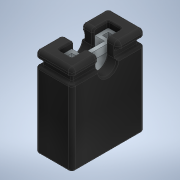
# Autodesk Inventor part: PinHeaderJumper
Saved by Autodesk Inventor 2021 (Build 250183000, 183)
## iProperties
Created: 2021-09-29
Part Number: PinHeaderJumper
Material: Generic
Document SubType Name: Modeling
Designer: ermoz
Density: 1 g/cm^3
Appearance: Default
Author: ermoz
Autodesk Inventor part; units mm, degrees
ref_plane "YZ Plane" through (0, 0, 0) normal (1, 0, 0) x (0, 1, 0)
sketch "Sketch1" plane through (0, 0, 0) normal (0, 1, 0) x (-1, 0, 0)
  line L0 (1.27, 2.54) -> (-1.27, 2.54)
  line L1 (-1.27, 2.54) -> (-1.27, -2.54)
  line L2 (-1.27, -2.54) -> (1.27, -2.54)
  line L3 (1.27, -2.54) -> (1.27, 2.54)
  line L4 (1.27, 2.54) -> (-1.27, -2.54) construction
  line L5 (-1.27, 2.54) -> (1.27, -2.54) construction
  line L6 (0.47, 1.74) -> (-0.47, 1.74)
  line L7 (-0.47, 1.74) -> (-0.47, -1.74)
  line L8 (-0.47, -1.74) -> (0.47, -1.74)
  line L9 (0.47, -1.74) -> (0.47, 1.74)
  point P0 (0, 0)
  dimension "d0" = 2.54
  dimension "d1" = 5.08
  dimension "d2" = 0.8
  constraints: 20 end point, 4 parallel, 2 midpoint, 2 perpendicular, 1 horizontal, 3 other
  measures "d0" distance of L2.end L1.end
  measures "d1" distance of L0.end L1.end
  measures "d2" distance between parallel lines of L3 L9
extrude "Extrusion1" add sketch "Sketch1" along normal blind 6.2
sketch "Sketch2" plane through (1.27, 0, 2.54) normal (1, 0, 0) x (0, 0, -1)
  line L0 (3.19, 5.2) -> (1.89, 5.2)
  line L1 (1.89, 5.2) -> (1.89, 7.2)
  line L2 (1.89, 7.2) -> (3.19, 7.2)
  line L3 (3.19, 7.2) -> (3.19, 5.2)
  line L4 (0, 6.2) -> (5.08, 6.2) projected
  line L5 (3.19, 5.2) -> (1.89, 7.2) construction
  line L6 (1.89, 5.2) -> (3.19, 7.2) construction
  circle A0 centre (2.54, 5.2) radius 0.65
  point P0 (2.54, 0)
  point P1 (2.54, 6.2)
  point P2 (3.19, 6.2)
  point P3 (1.89, 6.2)
  dimension "d5" = 1.3
  dimension "d6" = 2
  constraints: 12 end point, 4 midpoint, 2 parallel, 1 horizontal, 1 perpendicular, 3 other
  measures "d5" distance of L1.end L2.end
  measures "d6" distance of L2.end L0.start
extrude "Extrusion2" cut sketch "Sketch2" against normal through all contours A0 L0 | A0 L1 L4 L3 | L0 A0
ref_plane "Work Plane1" through (0, 5.7, 0) normal (0, 1, 0) x (1, 0, 0)
sketch "Sketch3" plane through (0, 5.7, 0) normal (0, 1, 0) x (1, 0, 0)
  line L0 (1.27, -2.54) -> (1.27, -0.65) projected
  line L1 (-1.27, -2.54) -> (1.27, -2.54) projected
  line L2 (1.27, 2.54) -> (-1.27, 2.54) projected
  line L3 (-1.27, 2.54) -> (1.27, 2.54)
  line L4 (1.27, 2.54) -> (1.27, -2.54)
  line L5 (1.27, -2.54) -> (-1.27, -2.54)
  line L6 (-1.27, -2.54) -> (-1.27, 2.54)
  line L7 (1.02, -2.29) -> (1.02, 2.29)
  line L8 (1.02, 2.29) -> (-1.02, 2.29)
  line L9 (-1.02, 2.29) -> (-1.02, -2.29)
  line L10 (-1.02, -2.29) -> (1.02, -2.29)
  point P0 (0, 0)
  dimension "d10" = 0.25
  constraints: 16 end point, 4 parallel, 2 perpendicular, 1 horizontal, 3 other
  measures "d10" distance between parallel lines of L4 L7
extrude "Extrusion3" cut sketch "Sketch3" against normal blind 0.5
fillet "Fillet1" radius 0.25 22 edges at (1.27, 6.2, 1.595) (0, 6.2, 2.54) (1.27, 5.95, 2.54) (1.27, 2.6, 2.54) (-1.27, 2.6, 2.54) (-1.27, 5.95, 2.54) (-1.27, 6.2, 1.595) (-1.27, 6.2, -1.595) (-1.27, 5.95, -2.54) (-1.27, 2.6, -2.54) (0, 6.2, -2.54) (1.27, 5.95, -2.54) (1.27, 2.6, -2.54) (1.27, 6.2, -1.595) (0.87, 6.2, -0.65) (1.27, 5.95, -0.65) (-1.27, 5.95, -0.65) (-0.87, 6.2, -0.65) (1.27, 5.95, 0.65) (0.87, 6.2, 0.65) (-1.27, 5.95, 0.65) (-0.87, 6.2, 0.65)
fillet "Fillet2" radius 0.1 32 edges at (-0.47, 6.1268, 0.7232) (-0.47, 5.575, 0.65) (-0.47, 4.55, 0) (-0.47, 5.575, -0.65) (-0.47, 6.1268, -0.7232) (-0.47, 6.2, -1.32) (-0.47, 6.2, 1.32) (0, 6.2, 1.74) (-0.47, 3.1, 1.74) (-0.47, 3.1, -1.74) (0, 6.2, -1.74) (0.47, 6.1268, -0.7232) (0.47, 5.575, -0.65) (0.47, 4.55, 0) (0.47, 5.575, 0.65) (0.47, 6.1268, 0.7232) (0.47, 6.2, 1.32) (0.47, 6.2, -1.32) (0.47, 3.1, -1.74) (0.47, 3.1, 1.74) (1.1968, 0, -2.4668) (0, 0, -2.54) (-1.1968, 0, -2.4668) (-1.27, 0, 0) (-1.1968, 0, 2.4668) (0, 0, 2.54) (1.1968, 0, 2.4668) (1.27, 0, 0) (0, 0, 1.74) (0.47, 0, 0) (-0.47, 0, 0) (0, 0, -1.74)
fillet "Fillet3" radius 0.1 42 edges at (1.1968, 5.2, -2.4668) (0, 5.2, -2.54) (-1.1968, 5.2, -2.4668) (-1.27, 5.2, -1.47) (1.27, 5.2, -1.47) (1.02, 5.2, -1.47) (0, 5.2, -2.29) (1.02, 5.45, -2.29) (-1.02, 5.2, -1.47) (-1.02, 5.45, -2.29) (0, 5.7, -2.29) (1.02, 5.7, -1.47) (-1.02, 5.7, -1.47) (-1.02, 5.7, 1.47) (-1.02, 5.2, 1.47) (-1.1968, 5.2, 2.4668) (0, 5.2, 2.54) (1.1968, 5.2, 2.4668) (1.27, 5.2, 1.47) (-1.27, 5.2, 1.47) (-1.02, 5.45, 2.29) (0, 5.2, 2.29) (0, 5.7, 2.29) (1.02, 5.45, 2.29) (1.02, 5.2, 1.47) (1.02, 5.7, 1.47) (1.1968, 5.7, 0.7232) (1.1968, 5.7, 2.4668) (0, 5.7, 2.54) (-1.1968, 5.7, 2.4668) (-1.27, 5.7, 1.595) (-1.1968, 5.7, 0.7232) (1.27, 5.7, 1.595) (1.1968, 5.7, -2.4668) (0, 5.7, -2.54) (-1.1968, 5.7, -2.4668) (-1.27, 5.7, -1.595) (-1.1968, 5.7, -0.7232) (1.1968, 5.7, -0.7232) (1.27, 5.7, -1.595) (-1.27, 4.55, 0) (1.27, 4.55, 0)
ref_plane "Work Plane2" through (0, 1, 0) normal (0, -1, 0) x (1, 0, 0)
sketch "Sketch4" plane through (0, 1, 0) normal (0, -1, 0) x (1, 0, 0)
  arc A0 (-0.47, -1.64) -> (-0.37, -1.74) centre (-0.37, -1.64) ccw projected
  line L0 (0.37, -1.74) -> (-0.37, -1.74) projected
  arc A1 (0.37, -1.74) -> (0.47, -1.64) centre (0.37, -1.64) ccw projected
  line L1 (0.47, 1.64) -> (0.47, -1.64) projected
  arc A2 (0.47, 1.64) -> (0.37, 1.74) centre (0.37, 1.64) ccw projected
  line L2 (-0.37, 1.74) -> (0.37, 1.74) projected
  arc A3 (-0.37, 1.74) -> (-0.47, 1.64) centre (-0.37, 1.64) ccw projected
  line L3 (-0.47, -1.64) -> (-0.47, 1.64) projected
  line L4 (-0.2, -1.47) -> (0.2, -1.47)
  line L5 (0.2, -1.47) -> (0.2, -1.07)
  line L6 (0.2, -1.07) -> (-0.2, -1.07)
  line L7 (-0.2, -1.07) -> (-0.2, -1.47)
  line L8 (-0.2, -1.47) -> (0.2, -1.07) construction
  line L9 (0.2, -1.47) -> (-0.2, -1.07) construction
  line L10 (-0.2, 1.07) -> (0.2, 1.07)
  line L11 (0.2, 1.07) -> (0.2, 1.47)
  line L12 (0.2, 1.47) -> (-0.2, 1.47)
  line L13 (-0.2, 1.47) -> (-0.2, 1.07)
  line L14 (-0.2, 1.07) -> (0.2, 1.47) construction
  line L15 (0.2, 1.07) -> (-0.2, 1.47) construction
  line L16 (0.2, -1.07) -> (0.2, 1.07)
  line L17 (0.47, -0.8) -> (-0.47, -0.8)
  line L18 (-0.47, -0.8) -> (-0.47, -1.74)
  line L19 (-0.47, -1.74) -> (0.47, -1.74)
  line L20 (0.47, -1.74) -> (0.47, -0.8)
  line L21 (0.47, -0.8) -> (-0.47, -1.74) construction
  line L22 (-0.47, -0.8) -> (0.47, -1.74) construction
  line L23 (0.47, 0.8) -> (-0.47, 0.8)
  line L24 (-0.47, 0.8) -> (-0.47, 1.74)
  line L25 (-0.47, 1.74) -> (0.47, 1.74)
  line L26 (0.47, 1.74) -> (0.47, 0.8)
  line L27 (0.47, 0.8) -> (-0.47, 1.74) construction
  line L28 (-0.47, 0.8) -> (0.47, 1.74) construction
  point P0 (0, 0)
  point P1 (0, -1.27)
  point P2 (0, 1.27)
  point P3 (0.2, 0.8)
  point P4 (0.2, -0.8)
  dimension "d17" = 0.4
  dimension "d18" = 0.4
  dimension "d19" = 0.4
  dimension "d20" = 0.4
  dimension "d21" = 2.54
  dimension "d22" = 1.27
  constraints: 50 end point, 8 midpoint, 8 parallel, 4 horizontal, 4 perpendicular, 1 point on line, 1 vertical
  measures "d17" distance of L6.end L5.end
  measures "d18" distance of L5.end L4.end
  measures "d19" distance of L12.end L11.end
  measures "d20" distance of L11.end L10.end
  measures "d21" distance of point (0, 1.27) point (0, -1.27)
  measures "d22" distance of point (0, -1.27) point (0, 0)
extrude "Extrusion4" add sketch "Sketch4" against normal blind 4.75 separate body contours L3 L17 L1 A1 L0 A0 | L3 A3 L2 A2 L1 L23 | L16 L23 L1 L17
ref_plane "Work Plane3" through (0, 2, 0) normal (0, -1, 0) x (1, 0, 0)
sketch "Sketch5" plane through (0, 2, 0) normal (0, -1, 0) x (1, 0, 0)
  line L0 (0.2, 0.8) -> (0.2, -0.8) projected
  line L1 (0.2, -0.8) -> (0.47, -0.8)
  line L2 (0.47, -0.8) -> (0.47, 0.8)
  line L3 (0.47, 0.8) -> (0.2, 0.8)
  line L4 (0.2, 0.8) -> (0.2, -0.8)
  line L5 (0.2, 0.8) -> (-0.47, 0.8) projected
  line L6 (0.47, 1.64) -> (0.47, -1.64) projected
  point P0 (0, 0)
  constraints: 8 end point, 2 collinear, 2 parallel, 1 horizontal, 1 perpendicular
extrude "Extrusion5" cut sketch "Sketch5" against normal blind 3.25 bodies 2
body "Solid1"
body "Solid2"
